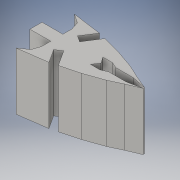
# Autodesk Inventor part: Part1
Saved by Autodesk Inventor 2016 (Build 200138000, 138)
## iProperties
Created: 2017-09-13
Part Number: Part1
Material: Generic
Document SubType Name: Modeling
Designer: student
Density: 1 g/cm^3
Appearance: Default
Author: student
Autodesk Inventor part; units mm, degrees
ref_plane "YZ Plane" through (0, 0, 0) normal (1, 0, 0) x (0, 1, 0)
ref_plane "XZ Plane" through (0, 0, 0) normal (0, 1, 0) x (-1, 0, 0)
ref_plane "XY Plane" through (0, 0, 0) normal (0, 0, 1) x (1, 0, 0)
sketch "Sketch1" plane through (0, 0, 0) normal (0, 1, 0) x (-1, 0, 0)
  line L0 (-17.4285, 2.7736) -> (-12.1383, 5.2631)
  line L1 (-12.1383, 5.2631) -> (-3.84, 8.1675)
  line L2 (-3.84, 8.1675) -> (4.2592, 10.3027)
  line L3 (7.5702, 11.1757) -> (20.3289, 12.9391)
  line L4 (20.3289, 12.9391) -> (16.3872, 10.2421)
  line L5 (16.3872, 10.2421) -> (15.2462, 6.7153)
  line L6 (15.2462, 6.7153) -> (15.2462, 2.676)
  line L7 (15.2462, 2.676) -> (24.4575, 2.676)
  line L8 (24.4575, 2.676) -> (24.4575, 0)
  line L9 (-17.4285, 2.7736) -> (-23.3511, 0.2916)
  line L10 (24.4575, 0) -> (-4.2928, 0)
  line L11 (-17.4285, -2.7736) -> (-12.1383, -5.2631)
  line L12 (-12.1383, -5.2631) -> (-3.84, -8.1675)
  line L13 (-3.84, -8.1675) -> (4.2592, -10.3027)
  line L14 (7.5702, -11.1757) -> (20.3289, -12.9391)
  line L15 (20.3289, -12.9391) -> (16.3872, -10.2421)
  line L16 (16.3872, -10.2421) -> (15.2462, -6.7153)
  line L17 (15.2462, -6.7153) -> (15.2462, -2.676)
  line L18 (15.2462, -2.676) -> (24.4575, -2.676)
  line L19 (24.4575, -2.676) -> (24.4575, 0)
  line L20 (-17.4285, -2.7736) -> (-23.3511, -0.2916)
  line L21 (15.2462, -2.676) -> (15.2462, 2.676)
  line L22 (7.5702, 11.1757) -> (11.3708, 5.2631)
  line L23 (11.3708, 5.2631) -> (8.6308, 3.5018)
  line L24 (8.6308, 3.5018) -> (4.2592, 10.3027)
  line L25 (7.5702, -11.1757) -> (11.3708, -5.2631)
  line L26 (8.6308, -3.5018) -> (4.2592, -10.3027)
  line L27 (11.3708, -5.2631) -> (8.6308, -3.5018)
  line L28 (-9.2958, -1.5896) -> (-6.6168, -2.7736)
  line L29 (-6.6168, -2.7736) -> (-2.4179, -2.7736)
  line L30 (-2.4179, -2.7736) -> (-4.2928, 0)
  line L31 (-9.2958, 1.5896) -> (-6.6168, 2.7736)
  line L32 (-6.6168, 2.7736) -> (-2.4179, 2.7736)
  line L33 (-2.4179, 2.7736) -> (-4.2928, 0)
  line L34 (-9.2958, 1.5896) -> (-16.9323, 1.5896)
  line L35 (-23.3511, 0.2916) -> (-16.9323, 1.5896)
  line L36 (-9.2958, -1.5896) -> (-16.9323, -1.5896)
  line L37 (-23.3511, -0.2916) -> (-16.9323, -1.5896)
  point P0 (0, 0)
  point P1 (0, 0)
  constraints: 76 end point, 17 symmetric about line, 4 perpendicular, 1 collinear, 1 horizontal
extrude "Extrusion1" add sketch "Sketch1" along normal blind 25.4
body "Solid1"
